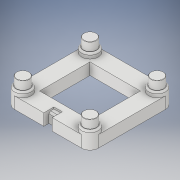
# Autodesk Inventor part: Bauteil2
Saved by Autodesk Inventor 2019.5 (Build 235369000, 369)
## iProperties
Created: 2021-09-27
Part Number: Bauteil2
Material: ABS-Kunststoff
Document SubType Name: Modeling
Designer: mritt
Density: 1.06 g/cm^3
Appearance: Glatt - Weiß
Mass: 6.54291 g
Surface Area: 47.1556 cm^2
Volume: 6.17256 cm^3
Author: mritt
Autodesk Inventor part; units mm, degrees
ref_plane "YZ Plane" through (0, 0, 0) normal (1, 0, 0) x (0, 1, 0)
ref_plane "XZ Plane" through (0, 0, 0) normal (0, 1, 0) x (-1, 0, 0)
ref_plane "XY Plane" through (0, 0, 0) normal (0, 0, 1) x (1, 0, 0)
sketch "Skizze1" plane through (0, 0, 0) normal (0, 1, 0) x (-1, 0, 0)
  line L0 (22.2037, -3.3333) -> (4.7037, -3.3333)
  line L1 (4.7037, -3.3333) -> (4.7037, -43.3333)
  line L2 (4.7037, -43.3333) -> (22.2037, -43.3333)
  line L3 (22.2037, -43.3333) -> (22.2037, -3.3333)
  circle A0 centre (14.7037, -10.0279) radius 3.75
  circle A1 centre (13.4537, -34.7142) radius 3.75
  line L4 (96.8973, -70.154) -> (56.8973, -70.154)
  line L5 (56.8973, -70.154) -> (56.8973, -110.154)
  line L6 (56.8973, -110.154) -> (96.8973, -110.154)
  line L7 (96.8973, -110.154) -> (96.8973, -70.154)
  circle A2 centre (96.8973, -110.154) radius 5
  circle A3 centre (56.8973, -110.154) radius 5
  circle A4 centre (56.8973, -70.154) radius 5
  circle A5 centre (96.8973, -70.154) radius 5
  circle A6 centre (96.8973, -70.154) radius 3.75
  circle A7 centre (96.8973, -110.154) radius 3.75
  circle A8 centre (56.8973, -70.154) radius 3.75
  circle A9 centre (56.8973, -110.154) radius 3.75
  line L8 (96.8973, -65.154) -> (56.8973, -65.154)
  line L9 (56.8973, -65.154) -> (56.8973, -75.154)
  line L10 (56.8973, -75.154) -> (96.8973, -75.154)
  line L11 (96.8973, -75.154) -> (96.8973, -65.154)
  line L12 (56.8973, -115.154) -> (96.8973, -115.154)
  line L13 (101.8973, -110.154) -> (101.8973, -70.154)
  line L14 (91.8973, -70.154) -> (91.8973, -110.154)
  line L15 (96.8973, -105.154) -> (56.8973, -105.154)
  line L16 (51.8973, -70.154) -> (51.8973, -110.154)
  line L17 (61.8973, -70.154) -> (61.8973, -110.154)
  line L18 (51.8973, -96.8467) -> (53.9203, -96.8467)
  line L19 (53.9203, -96.8467) -> (53.9203, -88.3797)
  line L20 (53.9203, -88.3797) -> (51.8973, -88.3797)
  line L21 (51.8973, -88.3797) -> (51.8973, -96.8467)
  point P0 (0, 0)
  dimension "d0" = 40
  dimension "d1" = 7.5
  dimension "d2" = 7.5
  dimension "d4" = 8.75
  dimension "d5" = 7.5
  dimension "d6" = 8.75
  dimension "d7" = 40
  dimension "d8" = 40
  dimension "d9" = 10
  dimension "d10" = 10
  dimension "d11" = 10
  dimension "d12" = 10
  dimension "d13" = 7.5
  dimension "d14" = 7.5
  dimension "d15" = 7.5
  dimension "d16" = 7.5
  dimension "d17" = 5
  dimension "d18" = 5
  dimension "d33" = 40
  constraints: 44 end point, 12 point on circle, 10 centre point, 8 coincident, 8 parallel, 8 point on line, 4 horizontal, 4 perpendicular, 4 tangent
  measures "d0" distance of L2.end L0.start
  measures "d1" diameter of A0
  measures "d2" diameter of A1
  measures "d4" distance from line of L3 A1.centre
  measures "d5" distance from line of L3 A0.centre
  measures "d6" distance from line of L1 A1.centre
  measures "d7" distance of L5.end L6.end
  measures "d8" distance of L6.end L4.start
  measures "d9" diameter of A5
  measures "d10" diameter of A2
  measures "d11" diameter of A3
  measures "d12" diameter of A4
  measures "d13" diameter of A6
  measures "d14" diameter of A7
  measures "d15" diameter of A9
  measures "d16" diameter of A8
  measures "d17" distance between parallel lines of L4 L8
  measures "d18" distance between parallel lines of L4 L10
  measures "d33" distance of L9.end L10.end
extrude "Extrusion1" add sketch "Skizze1" along normal blind 10 contours A6 L11 L4 | L4 L7 A6 | A8 L5 L4 | L4 L9 A8 | L11 A6 L7 | L5 A8 L9 | A7 L6 L7 | L7 L6 A7 | A9 L6 L5 | L5 L6 A9
extrude "Extrusion2" add sketch "Skizze1" along normal blind 5 contours A5 L11 A6 L4 | L4 A6 L7 A5 | A4 L5 A8 L4 | L4 A8 L9 A4 | A5 L7 A6 L11 | L9 A8 L5 A4 | A2 L6 A7 L7 | L7 A7 L6 A2 | A3 L6 A9 L5 | L5 A9 L6 A3
extrude "Extrusion4" add sketch "Skizze1" along normal blind 2 and the other way blind 5 contours L14 L10 L17 L4 | A5 L11 A6 L4 | L4 A4 L8 A5 | L4 A6 L7 A5 | A5 L10 L14 | A4 L5 A8 L4 | L4 A8 L9 A4 | L17 L10 A4 | A6 L11 L4 | L4 L7 A6 | A5 L7 A6 L11 | A5 L13 A2 L7 | L7 L15 L14 L10 | A8 L5 L4 | L4 L9 A8 | L9 A8 L5 A4 | L10 L17 L15 L5 | L5 A3 L16 L18 L19 L20 A4 | L11 A6 L7 | A2 L6 A7 L7 | L7 A7 L6 A2 | A2 L14 L15 | L14 L6 L17 L15 | L5 A8 L9 | A3 L6 A9 L5 | L15 L17 A3 | L5 A9 L6 A3 | A7 L6 L7 | L7 L6 A7 | A2 L12 A3 L6 | L20 L19 L18 L16 | A9 L6 L5 | L5 L6 A9
fillet "Rundung2" radius 1 4 edges at (-51.8973, 5, -110.154) (-91.8973, 5, -110.154) (-91.8973, 5, -70.154) (-51.8973, 5, -70.154)
fillet "Rundung3" radius 0.2 4 edges at (-93.1473, 10, -70.154) (-93.1473, 10, -110.154) (-53.1473, 10, -70.154) (-53.1473, 10, -110.154)
sketch "Skizze2" plane through (0, -5, 0) normal (0, -1, 0) x (1, 0, 0)
  line L0 (-56.8973, -65.154) -> (-96.8973, -65.154) projected
  line L1 (-79.3973, -65.154) -> (-74.3973, -65.154)
  line L2 (-74.3973, -65.154) -> (-74.3973, -68.154)
  line L3 (-74.3973, -68.154) -> (-79.3973, -68.154)
  line L4 (-79.3973, -68.154) -> (-79.3973, -65.154)
  point P0 (0, 0)
  dimension "d42" = 17.5
  dimension "d43" = 5
  dimension "d44" = 3
  constraints: 8 end point, 2 parallel, 1 horizontal, 1 perpendicular, 1 point on line
  measures "d42" distance from line of L4 L0.end
  measures "d43" distance of L2.end L3.end
  measures "d44" distance of L1.end L2.end
sketch "Skizze3" plane through (0, 2, 0) normal (0, 1, 0) x (1, 0, 0)
  line L0 (-74.3973, 68.154) -> (-79.3973, 68.154) projected
  line L1 (-74.3973, 68.154) -> (-79.3973, 68.154)
  line L2 (-79.3973, 68.154) -> (-79.3973, 71.154)
  line L3 (-79.3973, 71.154) -> (-74.3973, 71.154)
  line L4 (-74.3973, 71.154) -> (-74.3973, 68.154)
  point P0 (0, 0)
  dimension "d47" = 3
  constraints: 8 end point, 2 parallel, 1 horizontal, 1 perpendicular
  measures "d47" distance of L1.end L2.end
extrude "Extrusion8" cut sketch "Skizze3" against normal blind 1
extrude "Extrusion9" cut sketch "Skizze2" against normal blind 10
chamfer "Fase3" distance 1 angle 45 1 edges at (-76.8973, 1, -68.154)
